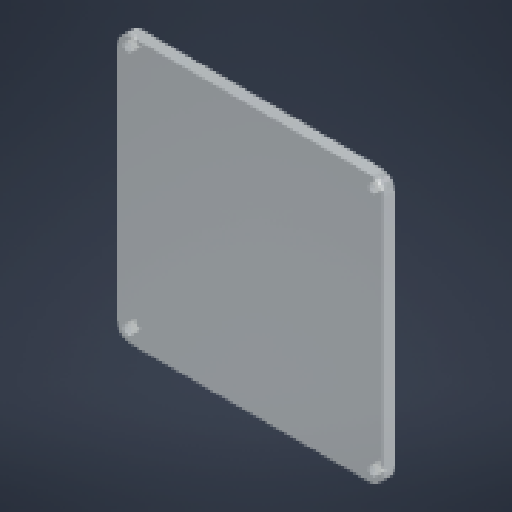
# Autodesk Inventor part: Protector_80x80
Saved by Autodesk Inventor 2024.1 (Build 281209000, 209)
## iProperties
Created: 2023-08-05
Part Number: Protector_80x80
Material: Glass
Document SubType Name: Modeling
Designer: jaege
Density: 2.18 g/cm^3
Appearance: Clear
Author: jaege
Autodesk Inventor part; units mm, degrees
ref_plane "YZ Plane" through (0, 0, 0) normal (1, 0, 0) x (0, 1, 0)
ref_plane "XZ Plane" through (0, 0, 0) normal (0, 1, 0) x (-1, 0, 0)
ref_plane "XY Plane" through (0, 0, 0) normal (0, 0, 1) x (1, 0, 0)
sketch "Sketch1" plane through (0, 0, 0) normal (0, 0, 1) x (1, 0, 0)
  line L0 (-40, 28) -> (40, 28) construction
  line L1 (-40, -52) -> (-40, 28) construction
  line L2 (-40, 53) -> (-40, 133) construction
  line L3 (-40, 133) -> (40, 133) construction
  line L4 (40, 133) -> (40, 53) construction
  line L5 (40, 53) -> (-40, 53) construction
  line L6 (-40, -52) -> (-40, 28) construction
  line L7 (-40, 28) -> (40, 28) construction
  line L8 (40, 28) -> (40, -52) construction
  line L9 (40, -52) -> (-40, -52) construction
  circle A0 centre (-27.5, 195) radius 1.5 construction
  circle A1 centre (27.5, 195) radius 1.5 construction
  circle A2 centre (27.5, -116) radius 1.5 construction
  circle A3 centre (-27.5, -116) radius 1.5 construction
  circle A4 centre (-27.5, -183) radius 1.5 construction
  circle A5 centre (27.5, -183) radius 1.5 construction
  line L10 (-37.5, -118) -> (-72.5, -118) construction
  line L11 (-72.5, -118) -> (-72.5, -114) construction
  line L12 (-72.5, -114) -> (-37.5, -114) construction
  line L13 (-37.5, -114) -> (-37.5, -118) construction
  line L14 (72.5, 197) -> (72.5, 193) construction
  line L15 (72.5, 193) -> (37.5, 193) construction
  line L16 (37.5, 193) -> (37.5, 197) construction
  line L17 (37.5, 197) -> (72.5, 197) construction
  line L18 (-17.5, 197) -> (17.5, 197) construction
  line L19 (17.5, 197) -> (17.5, 193) construction
  line L20 (17.5, 193) -> (-17.5, 193) construction
  line L21 (-17.5, 193) -> (-17.5, 197) construction
  line L22 (-37.5, -185) -> (-72.5, -185) construction
  line L23 (-72.5, -185) -> (-72.5, -181) construction
  line L24 (-72.5, -181) -> (-37.5, -181) construction
  line L25 (-37.5, -181) -> (-37.5, -185) construction
  line L26 (17.5, -118) -> (-17.5, -118) construction
  line L27 (-17.5, -118) -> (-17.5, -114) construction
  line L28 (-17.5, -114) -> (17.5, -114) construction
  line L29 (17.5, -114) -> (17.5, -118) construction
  line L30 (72.5, -185) -> (37.5, -185) construction
  line L31 (37.5, -185) -> (37.5, -181) construction
  line L32 (37.5, -181) -> (72.5, -181) construction
  line L33 (72.5, -181) -> (72.5, -185) construction
  line L34 (-37.5, 193) -> (-72.5, 193) construction
  line L35 (-72.5, 193) -> (-72.5, 197) construction
  line L36 (-72.5, 197) -> (-37.5, 197) construction
  line L37 (-37.5, 197) -> (-37.5, 193) construction
  line L38 (17.5, -181) -> (17.5, -185) construction
  line L39 (17.5, -185) -> (-17.5, -185) construction
  line L40 (-17.5, -185) -> (-17.5, -181) construction
  line L41 (-17.5, -181) -> (17.5, -181) construction
  line L42 (72.5, -114) -> (72.5, -118) construction
  line L43 (72.5, -118) -> (37.5, -118) construction
  line L44 (37.5, -118) -> (37.5, -114) construction
  line L45 (37.5, -114) -> (72.5, -114) construction
  circle A6 centre (-102, 39.5) radius 1.5 construction
  circle A7 centre (-102, -110.5) radius 1.5 construction
  circle A8 centre (102, -35.5) radius 1.5 construction
  circle A9 centre (102, 114.5) radius 1.5 construction
  circle A10 centre (102, -185.5) radius 1.5 construction
  circle A11 centre (-102, 189.5) radius 1.5 construction
  line L46 (100, 188) -> (95.2, 188) construction
  line L47 (95.2, 188) -> (95.2, 186.8) construction
  line L48 (95.2, 186.8) -> (92.8, 186.8) construction
  line L49 (92.8, 186.8) -> (92.8, 188) construction
  line L50 (92.8, 188) -> (88, 188) construction
  line L51 (88, 188) -> (88, 191) construction
  line L52 (88, 191) -> (92.8, 191) construction
  line L53 (92.8, 191) -> (92.8, 192.2) construction
  line L54 (92.8, 192.2) -> (95.2, 192.2) construction
  line L55 (95.2, 192.2) -> (95.2, 191) construction
  line L56 (95.2, 191) -> (100, 191) construction
  line L57 (100, 227) -> (100, 191) construction
  line L58 (87.5, 227) -> (100, 227) construction
  line L59 (87.5, 231) -> (87.5, 227) construction
  line L60 (52.5, 231) -> (87.5, 231) construction
  line L61 (52.5, 227) -> (52.5, 231) construction
  line L62 (36.5, 227) -> (52.5, 227) construction
  line L63 (36.5, 222.2) -> (36.5, 227) construction
  line L64 (37.7, 222.2) -> (36.5, 222.2) construction
  line L65 (37.7, 219.8) -> (37.7, 222.2) construction
  line L66 (36.5, 219.8) -> (37.7, 219.8) construction
  line L67 (36.5, 215) -> (36.5, 219.8) construction
  line L68 (33.5, 215) -> (36.5, 215) construction
  line L69 (33.5, 219.8) -> (33.5, 215) construction
  line L70 (32.3, 219.8) -> (33.5, 219.8) construction
  line L71 (32.3, 222.2) -> (32.3, 219.8) construction
  line L72 (33.5, 222.2) -> (32.3, 222.2) construction
  line L73 (33.5, 227) -> (33.5, 222.2) construction
  line L74 (17.5, 227) -> (33.5, 227) construction
  line L75 (17.5, 231) -> (17.5, 227) construction
  line L76 (-17.5, 231) -> (17.5, 231) construction
  line L77 (-17.5, 227) -> (-17.5, 231) construction
  line L78 (-33.5, 227) -> (-17.5, 227) construction
  line L79 (-33.5, 222.2) -> (-33.5, 227) construction
  line L80 (-32.3, 222.2) -> (-33.5, 222.2) construction
  line L81 (-32.3, 219.8) -> (-32.3, 222.2) construction
  line L82 (-33.5, 219.8) -> (-32.3, 219.8) construction
  line L83 (-33.5, 215) -> (-33.5, 219.8) construction
  line L84 (-36.5, 215) -> (-33.5, 215) construction
  line L85 (-36.5, 219.8) -> (-36.5, 215) construction
  line L86 (-37.7, 219.8) -> (-36.5, 219.8) construction
  line L87 (-37.7, 222.2) -> (-37.7, 219.8) construction
  line L88 (-36.5, 222.2) -> (-37.7, 222.2) construction
  line L89 (-36.5, 227) -> (-36.5, 222.2) construction
  line L90 (-52.5, 227) -> (-36.5, 227) construction
  line L91 (-52.5, 231) -> (-52.5, 227) construction
  line L92 (-87.5, 231) -> (-52.5, 231) construction
  line L93 (-87.5, 227) -> (-87.5, 231) construction
  line L94 (-104, 227) -> (-87.5, 227) construction
  line L95 (-104, 152) -> (-104, 227) construction
  line L96 (-100, 152) -> (-104, 152) construction
  line L97 (-100, 116) -> (-100, 152) construction
  line L98 (-100, 116) -> (-95.2, 116) construction
  line L99 (-95.2, 116) -> (-95.2, 117.2) construction
  line L100 (-95.2, 117.2) -> (-92.8, 117.2) construction
  line L101 (-92.8, 117.2) -> (-92.8, 116) construction
  line L102 (-92.8, 116) -> (-88, 116) construction
  line L103 (-88, 116) -> (-88, 113) construction
  line L104 (-88, 113) -> (-92.8, 113) construction
  line L105 (-92.8, 113) -> (-92.8, 111.8) construction
  line L106 (-92.8, 111.8) -> (-95.2, 111.8) construction
  line L107 (-95.2, 111.8) -> (-95.2, 113) construction
  line L108 (-95.2, 113) -> (-100, 113) construction
  line L109 (-100, 77) -> (-100, 113) construction
  line L110 (-104, 77) -> (-100, 77) construction
  line L111 (-104, 2) -> (-104, 77) construction
  line L112 (-100, 2) -> (-104, 2) construction
  line L113 (-100, -34) -> (-100, 2) construction
  line L114 (-100, -34) -> (-95.2, -34) construction
  line L115 (-95.2, -34) -> (-95.2, -32.8) construction
  line L116 (-95.2, -32.8) -> (-92.8, -32.8) construction
  line L117 (-92.8, -32.8) -> (-92.8, -34) construction
  line L118 (-92.8, -34) -> (-88, -34) construction
  line L119 (-88, -34) -> (-88, -37) construction
  line L120 (-88, -37) -> (-92.8, -37) construction
  line L121 (-92.8, -37) -> (-92.8, -38.2) construction
  line L122 (-92.8, -38.2) -> (-95.2, -38.2) construction
  line L123 (-95.2, -38.2) -> (-95.2, -37) construction
  line L124 (-95.2, -37) -> (-100, -37) construction
  line L125 (-100, -73) -> (-100, -37) construction
  line L126 (-104, -73) -> (-100, -73) construction
  line L127 (-104, -148) -> (-104, -73) construction
  line L128 (-100, -148) -> (-104, -148) construction
  line L129 (-100, -184) -> (-100, -148) construction
  line L130 (-100, -184) -> (-95.2, -184) construction
  line L131 (-95.2, -184) -> (-95.2, -182.8) construction
  line L132 (-95.2, -182.8) -> (-92.8, -182.8) construction
  line L133 (-92.8, -182.8) -> (-92.8, -184) construction
  line L134 (-92.8, -184) -> (-88, -184) construction
  line L135 (-88, -184) -> (-88, -187) construction
  line L136 (-88, -187) -> (-92.8, -187) construction
  line L137 (-92.8, -187) -> (-92.8, -188.2) construction
  line L138 (-92.8, -188.2) -> (-95.2, -188.2) construction
  line L139 (-95.2, -188.2) -> (-95.2, -187) construction
  line L140 (-95.2, -187) -> (-100, -187) construction
  line L141 (-100, -223) -> (-100, -187) construction
  line L142 (-87.5, -223) -> (-100, -223) construction
  line L143 (-87.5, -231) -> (-87.5, -223) construction
  line L144 (-52.5, -231) -> (-87.5, -231) construction
  line L145 (-52.5, -223) -> (-52.5, -231) construction
  line L146 (-36.5, -223) -> (-52.5, -223) construction
  line L147 (-36.5, -218.2) -> (-36.5, -223) construction
  line L148 (-37.7, -218.2) -> (-36.5, -218.2) construction
  line L149 (-37.7, -215.8) -> (-37.7, -218.2) construction
  line L150 (-36.5, -215.8) -> (-37.7, -215.8) construction
  line L151 (-36.5, -211) -> (-36.5, -215.8) construction
  line L152 (-33.5, -211) -> (-36.5, -211) construction
  line L153 (-33.5, -215.8) -> (-33.5, -211) construction
  line L154 (-32.3, -215.8) -> (-33.5, -215.8) construction
  line L155 (-32.3, -218.2) -> (-32.3, -215.8) construction
  line L156 (-33.5, -218.2) -> (-32.3, -218.2) construction
  line L157 (-33.5, -223) -> (-33.5, -218.2) construction
  line L158 (-17.5, -223) -> (-33.5, -223) construction
  line L159 (-17.5, -231) -> (-17.5, -223) construction
  line L160 (17.5, -231) -> (-17.5, -231) construction
  line L161 (17.5, -223) -> (17.5, -231) construction
  line L162 (33.5, -223) -> (17.5, -223) construction
  line L163 (33.5, -218.2) -> (33.5, -223) construction
  line L164 (32.3, -218.2) -> (33.5, -218.2) construction
  line L165 (32.3, -215.8) -> (32.3, -218.2) construction
  line L166 (33.5, -215.8) -> (32.3, -215.8) construction
  line L167 (33.5, -211) -> (33.5, -215.8) construction
  line L168 (36.5, -211) -> (33.5, -211) construction
  line L169 (36.5, -215.8) -> (36.5, -211) construction
  line L170 (37.7, -215.8) -> (36.5, -215.8) construction
  line L171 (37.7, -218.2) -> (37.7, -215.8) construction
  line L172 (36.5, -218.2) -> (37.7, -218.2) construction
  line L173 (36.5, -223) -> (36.5, -218.2) construction
  line L174 (52.5, -223) -> (36.5, -223) construction
  line L175 (52.5, -231) -> (52.5, -223) construction
  line L176 (87.5, -231) -> (52.5, -231) construction
  line L177 (87.5, -223) -> (87.5, -231) construction
  line L178 (104, -223) -> (87.5, -223) construction
  line L179 (104, -148) -> (104, -223) construction
  line L180 (100, -148) -> (104, -148) construction
  line L181 (100, -112) -> (100, -148) construction
  line L182 (100, -112) -> (95.2, -112) construction
  line L183 (95.2, -112) -> (95.2, -113.2) construction
  line L184 (95.2, -113.2) -> (92.8, -113.2) construction
  line L185 (92.8, -113.2) -> (92.8, -112) construction
  line L186 (92.8, -112) -> (88, -112) construction
  line L187 (88, -112) -> (88, -109) construction
  line L188 (88, -109) -> (92.8, -109) construction
  line L189 (92.8, -109) -> (92.8, -107.8) construction
  line L190 (92.8, -107.8) -> (95.2, -107.8) construction
  line L191 (95.2, -107.8) -> (95.2, -109) construction
  line L192 (95.2, -109) -> (100, -109) construction
  line L193 (100, -73) -> (100, -109) construction
  line L194 (104, -73) -> (100, -73) construction
  line L195 (104, 2) -> (104, -73) construction
  line L196 (100, 2) -> (104, 2) construction
  line L197 (100, 38) -> (100, 2) construction
  line L198 (100, 38) -> (95.2, 38) construction
  line L199 (95.2, 38) -> (95.2, 36.8) construction
  line L200 (95.2, 36.8) -> (92.8, 36.8) construction
  line L201 (92.8, 36.8) -> (92.8, 38) construction
  line L202 (92.8, 38) -> (88, 38) construction
  line L203 (88, 38) -> (88, 41) construction
  line L204 (88, 41) -> (92.8, 41) construction
  line L205 (92.8, 41) -> (92.8, 42.2) construction
  line L206 (92.8, 42.2) -> (95.2, 42.2) construction
  line L207 (95.2, 42.2) -> (95.2, 41) construction
  line L208 (95.2, 41) -> (100, 41) construction
  line L209 (100, 77) -> (100, 41) construction
  line L210 (104, 77) -> (100, 77) construction
  line L211 (104, 152) -> (104, 77) construction
  line L212 (100, 152) -> (104, 152) construction
  line L213 (100, 188) -> (100, 152) construction
  line L214 (-40, 28) -> (40, 28) construction
  line L215 (40, 28) -> (40, -52) construction
  line L216 (40, -52) -> (-40, -52) construction
  line L217 (-40, -52) -> (-40, 28) construction
  line L218 (-41.0465, 34.0465) -> (41.0465, 34.0465)
  line L219 (46.0465, 29.0465) -> (46.0465, -53.0465)
  line L220 (41.0465, -58.0465) -> (-41.0465, -58.0465)
  line L221 (-46.0465, -53.0465) -> (-46.0465, 29.0465)
  circle A12 centre (-42.291, 30.291) radius 1.5
  line L222 (-40, 28) -> (40, -52) construction
  line L223 (-40, 28) -> (-46.0465, 34.0465) construction
  arc A13 (-41.0465, 34.0465) -> (-46.0465, 29.0465) centre (-41.0465, 29.0465) ccw
  arc A14 (46.0465, 29.0465) -> (41.0465, 34.0465) centre (41.0465, 29.0465) ccw
  arc A15 (41.0465, -58.0465) -> (46.0465, -53.0465) centre (41.0465, -53.0465) ccw
  arc A16 (-46.0465, -53.0465) -> (-41.0465, -58.0465) centre (-41.0465, -53.0465) ccw
  circle A17 centre (-42.291, -54.291) radius 1.5
  circle A18 centre (42.291, -54.291) radius 1.5
  circle A19 centre (42.291, 30.291) radius 1.5
  circle A20 centre (42.291, 50.709) radius 1.5 projected
  circle A21 centre (-42.291, -54.291) radius 1.5 projected
  circle A22 centre (42.291, 30.291) radius 1.5 projected
  circle A23 centre (42.291, 135.291) radius 1.5 projected
  circle A24 centre (-42.291, 50.709) radius 1.5 projected
  circle A25 centre (42.291, -54.291) radius 1.5 projected
  circle A26 centre (-42.291, 30.291) radius 1.5 projected
  circle A27 centre (-42.291, 135.291) radius 1.5 projected
  point P0 (0, 0)
  point P1 (0, -12)
  point P2 (-44.5821, 32.5821)
  dimension "d1" = 3
  dimension "d2" = 3.24
  dimension "d3" = 5
  dimension "d4" = 3.24
  dimension "d7" = 360
  constraints: 20 end point, 9 point on circle, 8 centre point, 8 tangent, 4 parallel, 3 equal radius, 2 perpendicular, 2 point on line, 1 collinear, 1 horizontal, 1 midpoint, 12 other
  measures "d1" diameter of A12
  measures "d2" distance of L0.start A12.centre
  measures "d3" radius of A13
  measures "d4" distance of point (-44.582, 32.582) A12.centre
extrude "Extrusion1" add sketch "Sketch1" along normal blind 4 contours L218 A14 L219 A15 L220 A16 L221 A13
body "Solid1"
